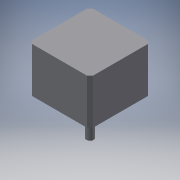
# Autodesk Inventor part: NEMA17
Saved by Autodesk Inventor 2016 (Build 200138000, 138)
## iProperties
Created: 2015-12-27
Part Number: NEMA17
Material: Generic
Document SubType Name: Modeling
Designer: inornate
Density: 1 g/cm^3
Appearance: Default
Author: inornate
Autodesk Inventor part; units mm, degrees
ref_plane "YZ Plane" through (0, 0, 0) normal (1, 0, 0) x (0, 1, 0)
ref_plane "XZ Plane" through (0, 0, 0) normal (0, 1, 0) x (-1, 0, 0)
ref_plane "XY Plane" through (0, 0, 0) normal (0, 0, 1) x (1, 0, 0)
sketch "Sketch1" plane through (0, 0, 0) normal (0, 0, 1) x (1, 0, 0)
  line L0 (19.9924, -21.8579) -> (16.7724, -25.0779) projected
  line L1 (19.9924, -21.8579) -> (19.9924, 20.4221) projected
  arc A0 (19.9924, 20.4221) -> (14.4924, 25.9221) centre (14.4924, 20.4221) ccw construction
  line L2 (14.4924, 25.9221) -> (14.2174, 25.9221) projected
  line L3 (14.2174, 25.9221) -> (14.2174, 26.4221) projected
  line L4 (9.7174, 30.9221) -> (14.2174, 26.4221) projected
  line L5 (-3.2826, 30.9221) -> (3.2174, 30.9221) projected
  line L6 (-7.7826, 26.4221) -> (-3.2826, 30.9221) projected
  line L7 (-7.7826, 25.9221) -> (-7.7826, 26.4221) projected
  line L8 (-7.7826, 25.9221) -> (-16.5076, 25.9221) projected
  arc A1 (-16.5076, 25.9221) -> (-22.0076, 20.4221) centre (-16.5076, 20.4221) ccw construction
  line L9 (-22.0076, 20.4221) -> (-22.0076, -10.5779) projected
  arc A2 (-22.0076, -10.5779) -> (-16.5076, -16.0779) centre (-16.5076, -10.5779) ccw construction
  line L10 (-16.5076, -16.0779) -> (-13.0076, -16.0779) projected
  line L11 (-13.0076, -16.0779) -> (-13.0076, -21.8579) projected
  line L12 (-9.7876, -25.0779) -> (-13.0076, -21.8579) projected
  line L13 (-9.7876, -25.0779) -> (-9.7826, -25.0779) projected
  line L14 (-12.7826, -28.0779) -> (-9.7826, -25.0779) projected
  line L15 (-15.5326, -28.0779) -> (-12.7826, -28.0779) projected
  line L16 (-15.5326, -28.0779) -> (-15.5326, -66.0779) projected
  arc A3 (-15.5326, -66.0779) -> (-9.5326, -72.0779) centre (-9.5326, -66.0779) ccw projected
  line L17 (-9.5326, -72.0779) -> (15.9674, -72.0779) projected
  arc A4 (15.9674, -72.0779) -> (21.9674, -66.0779) centre (15.9674, -66.0779) ccw projected
  line L18 (21.9674, -28.0779) -> (21.9674, -66.0779) projected
  line L19 (19.2174, -28.0779) -> (21.9674, -28.0779) projected
  line L20 (19.2174, -28.0779) -> (16.2174, -25.0779) projected
  line L21 (16.2174, -25.0779) -> (16.7724, -25.0779) projected
  circle A5 centre (-16.5076, 20.4221) radius 1.7 construction
  circle A6 centre (14.4924, 20.4221) radius 1.7 construction
  circle A7 centre (14.4924, -10.5779) radius 1.7 construction
  circle A8 centre (-16.5076, -10.5779) radius 1.7 construction
  circle A9 centre (14.7174, -41.5779) radius 2.25 projected
  circle A10 centre (-8.2826, -41.5779) radius 2.25 projected
  circle A11 centre (14.7174, -64.5779) radius 2.25 projected
  circle A12 centre (-8.2826, -64.5779) radius 2.25 projected
  circle A13 centre (-1.0076, 4.9221) radius 12.5 construction
  line L22 (-20.0076, 25.9221) -> (17.9924, 25.9221)
  line L23 (19.9924, 23.9221) -> (19.9924, -14.0779)
  line L24 (17.9924, -16.0779) -> (-20.0076, -16.0779)
  line L25 (-22.0076, -14.0779) -> (-22.0076, 23.9221)
  line L26 (-22.0076, 25.9221) -> (19.9924, -16.0779) construction
  line L27 (19.9924, 25.9221) -> (-22.0076, -16.0779) construction
  line L28 (-20.0076, 25.9221) -> (-22.0076, 23.9221)
  line L29 (17.9924, 25.9221) -> (19.9924, 23.9221)
  line L30 (19.9924, -14.0779) -> (17.9924, -16.0779)
  line L31 (-20.0076, -16.0779) -> (-22.0076, -14.0779)
  line L32 (7.7174, 40.9221) -> (8.8956, 39.0987) projected
  line L33 (5.2174, 40.9221) -> (7.7174, 40.9221) projected
  line L34 (3.2174, 38.9221) -> (5.2174, 40.9221) projected
  line L35 (3.2174, 30.9221) -> (3.2174, 38.9221) projected
  arc A14 (8.8956, 39.0987) -> (9.7174, 30.9221) centre (18.3776, 35.9221) ccw projected
  point P0 (0, 0)
  dimension "d0" = 2
  dimension "d1" = 2
  dimension "d2" = 2
  dimension "d3" = 2
  dimension "d4" = 2
  dimension "d5" = 2
  dimension "d6" = 2
  dimension "d7" = 2
  constraints: 20 end point, 10 point on line, 2 midpoint, 2 parallel, 1 horizontal, 1 perpendicular
  measures "d0" distance of L22.start L26.start
  measures "d1" distance of L25.end L26.start
  measures "d2" distance of L22.end L27.start
  measures "d3" distance of L23.start L27.start
  measures "d4" distance of L23.end L26.end
  measures "d5" distance of L24.start L26.end
  measures "d6" distance of L24.end L27.end
  measures "d7" distance of L25.start L27.end
extrude "Extrusion1" add sketch "Sketch1" along normal blind 31 contours L30 L24 L10 L31 L25 L9 L28 L22 L8 L2 L29 L23 L1
sketch "Sketch2" plane through (0, 0, 0) normal (0, 0, -1) x (-1, 0, 0)
  circle A0 centre (1.0076, 4.9221) radius 12.5 projected
  circle A1 centre (1.0076, 4.9221) radius 11
  point P0 (0, 0)
  dimension "d10" = 22
  constraints: 1 centre point, 1 coincident
  measures "d10" diameter of A1
extrude "Extrusion2" add sketch "Sketch2" along normal blind 2 contours A1
sketch "Sketch3" plane through (0, 0, 0) normal (0, 0, -1) x (-1, 0, 0)
  line L0 (20.0076, 25.9221) -> (22.0076, 23.9221) projected
  line L1 (-19.9924, 23.9221) -> (-17.9924, 25.9221) projected
  line L2 (-17.9924, -16.0779) -> (-19.9924, -14.0779) projected
  line L3 (22.0076, -14.0779) -> (20.0076, -16.0779) projected
  circle A0 centre (-14.4924, 20.4221) radius 1.5
  circle A1 centre (16.5076, 20.4221) radius 1.5
  line L4 (-18.9924, 24.9221) -> (21.0076, -15.0779) construction
  line L5 (21.0076, 24.9221) -> (-18.9924, -15.0779) construction
  circle A2 centre (-14.4924, -10.5779) radius 1.5
  circle A3 centre (16.5076, -10.5779) radius 1.5
  point P0 (0, 0)
  dimension "d13" = 31
  dimension "d14" = 3
  constraints: 4 centre point, 4 end point, 4 midpoint, 4 point on line, 3 equal radius, 2 vertical alignment, 1 horizontal alignment
  measures "d13" distance of A1.centre A0.centre
  measures "d14" diameter of A0
extrude "Extrusion3" cut sketch "Sketch3" against normal blind 5
sketch "Sketch4" plane through (-1.0076, 4.9221, -2) normal (0, 0, -1) x (-1, 0, 0)
  circle A0 centre (0, 0) radius 11 projected
  circle A1 centre (0, 0) radius 2.5
  point P0 (-1.0076, -4.9221)
  dimension "d17" = 5
  constraints: 1 centre point, 1 coincident
  measures "d17" diameter of A1
extrude "Extrusion4" add sketch "Sketch4" along normal blind 24 contours A1
equation "\"d1\" = d0"
equation "\"d2\" = d0"
equation "\"d3\" = d2"
equation "\"d4\" = d0"
equation "\"d5\" = d4"
equation "\"d6\" = d0"
equation "\"d7\" = d6"
body "Solid1"
